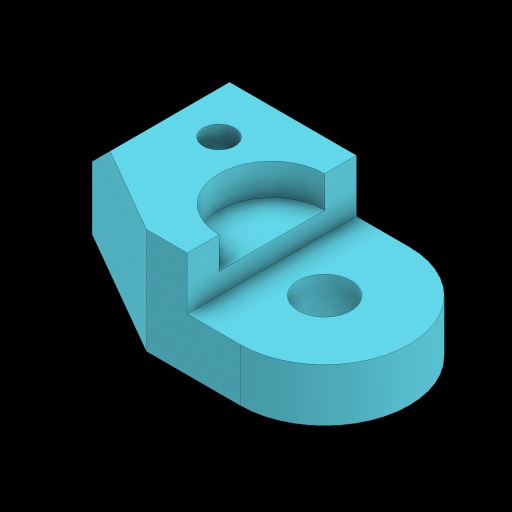
# Autodesk Inventor part: ANS8-2-BK
Saved by Autodesk Inventor 2024 (Build 280153000, 153)
## iProperties
Created: 2023-10-14
Part Number: ANS8-2-BK
Material: Bronze, Cast
Document SubType Name: Modeling
Designer: bennk
Density: 8.87 g/cm^3
Appearance: Cadet Blue
Mass: 6071.85 g
Surface Area: 634.153 cm^2
Volume: 684.537 cm^3
Author: bennk
Autodesk Inventor part; units mm, degrees
ref_plane "YZ Plane" through (0, 0, 0) normal (1, 0, 0) x (0, 1, 0)
ref_plane "XZ Plane" through (0, 0, 0) normal (0, 1, 0) x (-1, 0, 0)
ref_plane "XY Plane" through (0, 0, 0) normal (0, 0, 1) x (1, 0, 0)
sketch "Sketch1" plane through (0, 0, 0) normal (0, 1, 0) x (-1, 0, 0)
  circle A0 centre (0, 0) radius 15.875
  circle A1 centre (0, 0) radius 50.8
  line L0 (0, -50.8) -> (133.35, -50.8)
  line L1 (133.35, -50.8) -> (133.35, 6.35)
  line L2 (133.35, 6.35) -> (56.3603, 50.8)
  line L3 (56.3603, 50.8) -> (0, 50.8)
  circle A2 centre (82.55, -19.05) radius 9.525
  dimension "d0" = 101.6
  dimension "d1" = 133.35
  dimension "d4" = 60
  dimension "d5" = 57.15
  dimension "d6" = 31.75
  dimension "d7" = 19.05
  dimension "d8" = 31.75
  dimension "d9" = 82.55
  constraints: 8 end point, 3 centre point, 2 coincident, 2 horizontal, 2 point on circle, 2 tangent, 1 perpendicular
  measures "d0" diameter of A1
  measures "d1" distance of L0.start L0.end
  measures "d4" angle of L1 L2
  measures "d5" distance of L0.end L1.end
  measures "d6" diameter of A0
  measures "d7" diameter of A2
  measures "d8" distance from line of L0 A2.centre
  measures "d9" horizontal distance of point (0, 0) A2.centre
extrude "MAIN BLOCK" add sketch "Sketch1" along normal blind 63.5
sketch "Sketch2" plane through (0, 63.5, 0) normal (0, 1, 0) x (1, 0, 0)
  line L0 (-31.75, -50.8) -> (50.8, -50.8)
  line L1 (50.8, -50.8) -> (50.8, 50.8)
  line L2 (50.8, 50.8) -> (-31.75, 50.8)
  line L3 (-31.75, 50.8) -> (-31.75, -50.8)
  arc A0 (0, -50.8) -> (0, 50.8) centre (0, 0) ccw projected
  line L4 (0, 50.8) -> (-133.35, 50.8) projected
  line L5 (-56.3603, -50.8) -> (0, -50.8) projected
  point P0 (0, 50.8)
  dimension "d12" = 31.75
  constraints: 8 end point, 2 collinear, 2 parallel, 1 horizontal, 1 perpendicular, 1 tangent
  measures "d12" distance from line of point (0, 0) L3
extrude "SQUARE CUTOUT" cut sketch "Sketch2" against normal blind 31.75 contours L3 L2 A0 L0
sketch "Sketch3" plane through (0, 63.5, 0) normal (0, 1, 0) x (1, 0, 0)
  line L0 (-31.75, -50.8) -> (-31.75, 50.8) projected
  circle A0 centre (-31.75, 0) radius 31.75
  point P0 (0, 0)
  point P1 (-31.75, 31.75)
  point P2 (-31.75, -31.75)
  dimension "d15" = 63.5
  constraints: 1 centre point, 1 midpoint
  measures "d15" diameter of A0
extrude "HALF CIRCLE CUTOUT" cut sketch "Sketch3" against normal blind 19.05 contours A0 L0 picked at (-42.2562, -1.2757)
chamfer "REAR CHAMFER" distance 25.4 angle 45 1 edges at (-133.35, 63.5, -22.225)
body "Solid1"
